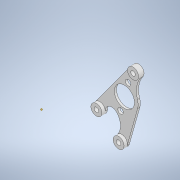
# Autodesk Inventor part: モータマウント
Saved by Autodesk Inventor 2022.2 (Build 262287010, 287A)
## iProperties
Created: 2022-01-29
Part Number: モータマウント
Material: Aluminum 2014-T4
Document SubType Name: Modeling
Designer: acps
Density: 2.8 g/cm^3
Appearance: Satin
Author: acps
Autodesk Inventor part; units mm, degrees
ref_plane "YZ Plane" through (0, 0, 0) normal (1, 0, 0) x (0, 1, 0)
ref_plane "XZ Plane" through (0, 0, 0) normal (0, 1, 0) x (-1, 0, 0)
ref_plane "XY Plane" through (0, 0, 0) normal (0, 0, 1) x (1, 0, 0)
sketch "Sketch1" plane through (0, 0, 0) normal (0, 0, 1) x (1, 0, 0)
  circle A0 centre (46.4683, 30) radius 5.5
  arc A1 (72.1609, 38.7902) -> (45.5671, 45.0103) centre (50.3015, 5.2915) ccw construction
  arc A2 (76.7854, 39.1678) -> (44.5539, 47.9057) centre (50.3015, 5.2915) ccw construction
  circle A3 centre (53.0056, 45.2) radius 1.25
  circle A4 centre (45.1, 8.5) radius 1.25
  circle A5 centre (48.5388, 37.7274) radius 1.5
  line L0 (48.5388, 37.7274) -> (46.4683, 30)
  line L1 (46.4683, 30) -> (44.3977, 22.2726)
  circle A6 centre (44.3977, 22.2726) radius 2.75 construction
  circle A7 centre (33, 18) radius 1.25
  arc A8 (53.6885, 27.9707) -> (53.6094, 32.2922) centre (46.4683, 30) ccw
  circle A9 centre (44.3977, 22.2726) radius 1.5
  circle A10 centre (53.0056, 45.2) radius 3
  circle A11 centre (33, 18) radius 3
  circle A12 centre (45.1, 8.5) radius 3
  arc A13 (55.4232, 43.4237) -> (53.6094, 32.2922) centre (65.4161, 36.0819) ccw
  arc A14 (42.7113, 10.315) -> (42.3368, 20.4518) centre (36.3415, 15.155) ccw
  arc A15 (42.3368, 20.4518) -> (35.9999, 18.0242) centre (39.6222, 18.0534) ccw
  line L2 (53.6885, 27.9707) -> (47.9881, 7.6883)
  line L3 (50.5889, 46.9775) -> (30.5833, 19.7775)
  line L4 (0, 0) -> (22.3079, 0) construction
  dimension "d29" = 5.5
  dimension "d24" = 11
  dimension "d25" = 3
  dimension "d26" = 3
  dimension "d27" = 8
  dimension "d28" = 8
  dimension "d31" = 2
  dimension "d32" = 3
  dimension "d34" = 6
  dimension "d35" = 6
  dimension "d36" = 6
  dimension "d39" = 12.4
  dimension "d45" = 8
  dimension "d46" = 105
  constraints: 18 point on circle, 15 centre point, 10 end point, 8 tangent, 7 coincident, 2 concentric, 1 collinear, 1 horizontal, 13 other
  measures "d24" diameter of A0
  measures "d25" radial gap between concentric circles of A2 A1
  measures "d26" diameter of A5
  measures "d27" distance of L0.start L0.end
  measures "d28" distance of L0.end L1.end
  measures "d31" radial gap between concentric circles of A8 A0
  measures "d32" diameter of A9
  measures "d34" diameter of A10
  measures "d35" diameter of A11
  measures "d36" diameter of A12
  measures "d39" radius of A13
  measures "d45" radius of A14
  measures "d46" angle of L4 L1
extrude "Extrusion1" add sketch "Sketch1" along normal blind 3 contours A12 | A10 | A11
extrude "Extrusion4" add sketch "Sketch1" along normal blind 1.2 contours L2 A12 A14 A15 A11 L3 A10 A13 A8
body "Solid1"
